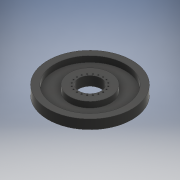
# Autodesk Inventor part: SG01
Saved by Autodesk Inventor 2017 (Build 210142000, 142)
## iProperties
Created: 2019-09-21
Part Number: SG01
Material: ABS Plastic
Document SubType Name: Modeling
Designer: Dell
Density: 1.06 g/cm^3
Appearance: Smooth - Black
Mass: 48.3343 g
Surface Area: 191.823 cm^2
Volume: 45.5984 cm^3
Author: Dell
Autodesk Inventor part; units mm, degrees
ref_plane "YZ Plane" through (0, 0, 0) normal (1, 0, 0) x (0, 1, 0)
ref_plane "XZ Plane" through (0, 0, 0) normal (0, 1, 0) x (-1, 0, 0)
ref_plane "XY Plane" through (0, 0, 0) normal (0, 0, 1) x (1, 0, 0)
sketch "Sketch1" plane through (0, 0, 0) normal (0, 0, 1) x (1, 0, 0)
  circle A0 centre (0, 0) radius 45
  circle A1 centre (0, 0) radius 12
  dimension "d0" = 90
  dimension "d1" = 24
  constraints: 2 centre point, 2 coincident
  measures "d0" diameter of A0
  measures "d1" diameter of A1
extrude "Extrusion1" add sketch "Sketch1" along normal blind 10
sketch "Sketch3" plane through (0, 0, 10) normal (0, 0, 1) x (1, 0, 0)
  circle A0 centre (20, 0) radius 1.75
  circle A1 centre (14.1421, 14.1421) radius 1.75
  circle A2 centre (0, 20) radius 1.75
  circle A3 centre (-14.1421, 14.1421) radius 1.75
  circle A4 centre (-20, 0) radius 1.75
  circle A5 centre (-14.1421, -14.1421) radius 1.75
  circle A6 centre (0, -20) radius 1.75
  circle A7 centre (14.1421, -14.1421) radius 1.75
  point P0 (0, 0)
  dimension "d13" = 3.5
  dimension "d14" = 20
  dimension "d17" = 360
  constraints: 8 centre point, 1 horizontal alignment, 17 other
  measures "d13" diameter of A0
  measures "d14" distance of A0.centre point (0, 0)
extrude "Extrusion3" [suppressed]
sketch "Sketch6" plane through (0, 0, 0) normal (0, 0, -1) x (-1, 0, 0)
  circle A0 centre (0, 14) radius 0.75
  circle A1 centre (-4.3262, 13.3148) radius 0.75
  circle A2 centre (-8.229, 11.3262) radius 0.75
  circle A3 centre (-11.3262, 8.229) radius 0.75
  circle A4 centre (-13.3148, 4.3262) radius 0.75
  circle A5 centre (-14, 0) radius 0.75
  circle A6 centre (-13.3148, -4.3262) radius 0.75
  circle A7 centre (-11.3262, -8.229) radius 0.75
  circle A8 centre (-8.229, -11.3262) radius 0.75
  circle A9 centre (-4.3262, -13.3148) radius 0.75
  circle A10 centre (0, -14) radius 0.75
  circle A11 centre (4.3262, -13.3148) radius 0.75
  circle A12 centre (8.229, -11.3262) radius 0.75
  circle A13 centre (11.3262, -8.229) radius 0.75
  circle A14 centre (13.3148, -4.3262) radius 0.75
  circle A15 centre (14, 0) radius 0.75
  circle A16 centre (13.3148, 4.3262) radius 0.75
  circle A17 centre (11.3262, 8.229) radius 0.75
  circle A18 centre (8.229, 11.3262) radius 0.75
  circle A19 centre (4.3262, 13.3148) radius 0.75
  point P0 (0, 0)
  dimension "d24" = 1.5
  dimension "d25" = 14
  dimension "d28" = 360
  constraints: 20 centre point, 1 vertical alignment, 41 other
  measures "d24" diameter of A0
  measures "d25" distance of A0.centre point (0, 0)
extrude "Extrusion5" cut sketch "Sketch6" against normal through all
sketch "Sketch7" plane through (0, 0, 10) normal (0, 0, 1) x (1, 0, 0)
  circle A0 centre (0, 0) radius 22
  circle A1 centre (0, 0) radius 38
  dimension "d32" = 44
  dimension "d33" = 76
  constraints: 2 centre point, 2 coincident
  measures "d32" diameter of A0
  measures "d33" diameter of A1
extrude "Extrusion6" cut sketch "Sketch7" against normal blind 6.35
body "Solid1"
